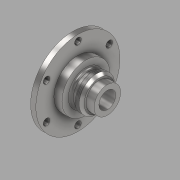
# Autodesk Inventor part: Lab15_A01209499
Saved by Autodesk Inventor 2020 (Build 240168000, 168)
## iProperties
Created: 2019-11-29
Part Number: Lab15_A01209499
Material: Acero, carbono
Document SubType Name: Modeling
Designer: Gerardo Naranjo
Density: 7.85 g/cm^3
Appearance: Semipulido
Project: Gerardo Naranjo
Engineer: Gerardo Naranjo
Author: Gerardo Naranjo
Title: Coupling
Autodesk Inventor part; units mm, degrees
ref_plane "YZ Plane" through (0, 0, 0) normal (1, 0, 0) x (0, 1, 0)
ref_plane "XZ Plane" through (0, 0, 0) normal (0, 1, 0) x (-1, 0, 0)
ref_plane "XY Plane" through (0, 0, 0) normal (0, 0, 1) x (1, 0, 0)
sketch "Boceto1" plane through (0, 0, 0) normal (0, 0, 1) x (1, 0, 0)
  line L0 (0, 0) -> (0, 50)
  line L1 (0, 50) -> (6.2, 50)
  line L2 (6.2, 50) -> (6.2, 28.5)
  line L3 (6.2, 28.5) -> (15.8, 28.5)
  line L4 (15.8, 28.5) -> (15.8, 21)
  line L5 (18.8, 18) -> (22.3, 18)
  line L6 (22.3, 18) -> (22.3, 21.9094) construction
  line L7 (41.2, 0) -> (0, 0)
  arc A0 (15.8, 21) -> (18.8, 18) centre (18.8, 21) ccw
  line L8 (22.3, 18) -> (28.4018, 18) construction
  line L9 (28.7, 21) -> (24.0321, 21)
  line L10 (22.3, 18) -> (24.0321, 21)
  line L11 (22.3, 18) -> (25.7641, 18) construction
  line L12 (59.327, 18) -> (29.2282, 18) construction
  line L13 (31.7, 18) -> (31.7, 21) construction
  line L14 (31.7, 18) -> (28.7, 21)
  line L15 (31.7, 18) -> (35.9426, 18) construction
  line L16 (31.7, 18) -> (41.2, 18) construction
  line L17 (41.2, 15.8) -> (41.2, 0)
  line L18 (31.7, 18) -> (31.7, 0)
  line L19 (31.7, 15.8) -> (41.2, 15.8)
  line L20 (22.3, 18) -> (22.3, 0)
  point P0 (15.8, 18)
  dimension "d0" = 50
  dimension "d1" = 6.2
  dimension "d2" = 9.6
  dimension "d3" = 28.5
  dimension "d4" = 6.5
  dimension "d5" = 3
  dimension "d8" = 18
  dimension "d10" = 21
  dimension "d11" = 60
  dimension "d12" = 18
  dimension "d14" = 9.4
  dimension "d15" = 135
  dimension "d16" = 9.5
  dimension "d17" = 41.2
  dimension "d18" = 15.8
  constraints: 42 end point, 9 perpendicular, 7 point on line, 6 horizontal, 3 vertical, 2 equal length, 2 point on circle, 2 tangent, 1 centre point
  measures "d0" distance of L0.start L0.end
  measures "d1" distance of L0.end L1.end
  measures "d2" distance of L2.end L3.end
  measures "d3" distance between parallel lines of L7 L3
  measures "d4" distance of point (15.8, 18) L5.end
  measures "d5" radius of A0
  measures "d8" distance between parallel lines of L7 L5
  measures "d10" distance between parallel lines of L7 L9
  measures "d11" angle of L11 L10
  measures "d12" distance between parallel lines of L7 L12
  measures "d14" distance between parallel lines of L6 L13
  measures "d15" angle of L15 L14
  measures "d16" distance of L13.start L16.end
  measures "d17" distance between parallel lines of L0 L17
  measures "d18" distance between parallel lines of L7 L19
revolve "Revolución1" add sketch "Boceto1" angle 360 about axis through (41.2, 0, 0) along (-1, 0, 0)
sketch "Boceto2" plane through (0, 0, 0) normal (-1, 0, 0) x (0, 0, 1)
  circle A0 centre (0, 0) radius 28.5 projected
  point P0 (0, 0)
  constraints: 1 coincident
hole "Agujero1" at (0, 0, 0) direction (1, 0, 0) diameter 20 end through all counterbore diameter 44.5 counterbore depth 9.5
sketch "Boceto3" plane through (0, 0, 0) normal (-1, 0, 0) x (0, 0, 1)
  point P0 (0, 0)
  point P1 (0, 43)
  point P2 (-37.2391, 21.5)
  point P3 (-37.2391, -21.5)
  point P4 (0, -43)
  point P5 (37.2391, -21.5)
  point P6 (37.2391, 21.5)
  dimension "d27" = 43
  dimension "d37" = 360
  constraints: 7 other
  measures "d27" distance of point (0, 0) point (0, 43)
hole "Agujero2" at (0, 43, 0) at (0, 21.5, 37.2391) at (0, -21.5, 37.2391) at (0, -43, 0) at (0, -21.5, -37.2391) at (0, 21.5, -37.2391) direction (1, 0, 0) diameter 7.9 end through all
thread "Rosca1" size "M42x1.5" class "6g" standard "ANSI Metric M Profile" full length
fillet "Empalme1" radius 2 1 edges at (9.5, 0, -22.25)
